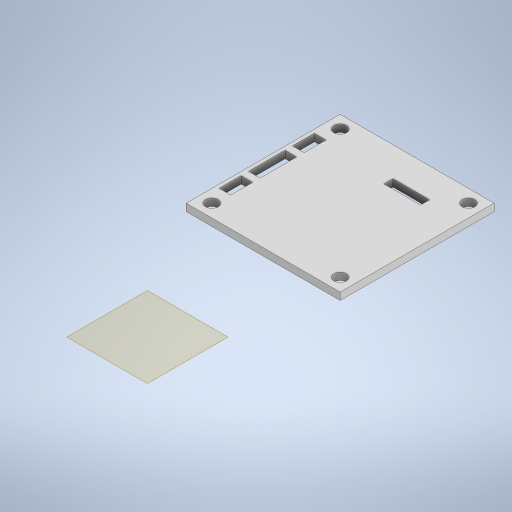
# Autodesk Inventor part: display_base
Saved by Autodesk Inventor 2023 (Build 270158000, 158)
## iProperties
Created: 2023-05-18
Part Number: display_base
Material: Generic
Document SubType Name: Modeling
Designer: mark
Density: 1 g/cm^3
Appearance: Default
Author: mark
Autodesk Inventor part; units mm, degrees
ref_plane "YZ Plane" through (0, 0, 0) normal (1, 0, 0) x (0, 1, 0)
ref_plane "XZ Plane" through (0, 0, 0) normal (0, 1, 0) x (-1, 0, 0)
ref_plane "XY Plane" through (0, 0, 0) normal (0, 0, 1) x (1, 0, 0)
ref_plane "Work Plane1" through (0, -2.5, 0) normal (0, 1, 0) x (1, 0, 0)
sketch "Sketch10" plane through (0, -2.5, 0) normal (0, 1, 0) x (1, 0, 0)
  line L0 (-24.3453, 76.929) -> (17.6547, 76.929)
  line L1 (17.6547, 76.929) -> (17.6547, 34.929)
  line L2 (17.6547, 34.929) -> (-24.3453, 34.929)
  line L3 (-24.3453, 34.929) -> (-24.3453, 76.929)
  circle A0 centre (-20.8453, 73.429) radius 1.75
  circle A1 centre (14.1547, 73.429) radius 1.75
  circle A2 centre (14.1547, 38.429) radius 1.75
  circle A3 centre (-20.8453, 38.429) radius 1.75
  line L4 (-23.3453, 68.929) -> (-20.1928, 68.929)
  line L5 (-20.1928, 68.929) -> (-20.1928, 42.929)
  line L6 (-20.1928, 42.929) -> (-23.3453, 42.929)
  line L7 (-24.3453, 42.929) -> (-24.3453, 68.9078)
  line L8 (-1.9453, 68.929) -> (8.0547, 68.929)
  line L9 (8.0547, 68.929) -> (8.0547, 66.429)
  line L10 (8.0547, 66.429) -> (-1.9453, 66.429)
  line L11 (-1.9453, 66.429) -> (-1.9453, 68.929)
  line L12 (-23.3453, 62.929) -> (-20.1928, 62.929)
  line L13 (-20.1928, 62.929) -> (-20.1928, 60.929)
  line L14 (-20.1928, 60.929) -> (-23.3453, 60.929)
  line L15 (-23.3453, 50.929) -> (-20.1928, 50.929)
  line L16 (-20.1928, 50.929) -> (-20.1928, 48.929)
  line L17 (-20.1928, 48.929) -> (-23.3453, 48.929)
  line L18 (-23.3453, 68.929) -> (-23.3453, 62.929)
  line L19 (-23.3453, 60.929) -> (-23.3453, 50.929)
  line L20 (-23.3453, 48.929) -> (-23.3453, 42.929)
  point P0 (0, 0)
  point P1 (8.0547, 67.679)
  point P2 (-21.769, 68.929)
  point P3 (-21.769, 62.929)
  point P4 (-21.769, 48.929)
  point P5 (-21.769, 50.929)
  point P6 (-21.769, 42.929)
  dimension "d76" = 42
  dimension "d77" = 42
  dimension "d78" = 3.5
  dimension "d79" = 3.5
  dimension "d80" = 3.5
  dimension "d81" = 3.5
  dimension "d82" = 3.5
  dimension "d83" = 3.5
  dimension "d84" = 3.5
  dimension "d85" = 3.5
  dimension "d86" = 3.5
  dimension "d88" = 10
  dimension "d89" = 2.5
  dimension "d90" = 8
  dimension "d91" = 9.6
  dimension "d92" = 6
  dimension "d93" = 2
  dimension "d94" = 2
  dimension "d95" = 6
  dimension "d96" = 8
  dimension "d97" = 8
  constraints: 42 end point, 8 parallel, 8 perpendicular, 6 midpoint, 5 horizontal, 4 centre point, 3 point on line
  measures "d76" distance of L1.end L2.end
  measures "d77" distance of L0.end L1.end
  measures "d78" diameter of A2
  measures "d79" distance from line of L0 A0.centre
  measures "d80" distance from line of L3 A0.centre
  measures "d81" distance from line of L0 A1.centre
  measures "d82" distance from line of L1 A1.centre
  measures "d83" distance from line of L1 A2.centre
  measures "d84" distance from line of L2 A2.centre
  measures "d85" distance from line of L2 A3.centre
  measures "d86" distance from line of L3 A3.centre
  measures "d88" distance of L9.end L10.end
  measures "d89" distance of L8.end L9.end
  measures "d90" distance between parallel lines of L0 L8
  measures "d91" distance from line of L1 point (8.055, 67.679)
  measures "d92" distance of point (-21.769, 68.929) point (-21.769, 62.929)
  measures "d93" distance from line of L12 L13.end
  measures "d94" distance of point (-21.769, 48.929) point (-21.769, 50.929)
  measures "d95" distance of point (-21.769, 42.929) point (-21.769, 48.929)
  measures "d96" distance from line of L0 L4.start
  measures "d97" distance from line of L2 L6.end
extrude "Extrusion9" add sketch "Sketch10" along normal blind 2
equation "\"d80\" = d79"
equation "\"d81\" = d80"
equation "\"d82\" = d80"
equation "\"d83\" = d80"
equation "\"d84\" = d83"
equation "\"d85\" = d80"
equation "\"d86\" = d80"
equation "\"d94\" = d93"
body "Solid1"
